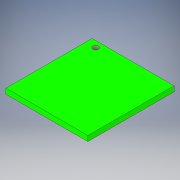
# Autodesk Inventor part: Vero_Board
Saved by Autodesk Inventor 2019.4 (Build 234330000, 330)
## iProperties
Created: 2021-06-29
Part Number: Vero_Board
Material: Generic
Document SubType Name: Modeling
Designer: keshav
Density: 1 g/cm^3
Appearance: Default
Author: keshav
Autodesk Inventor part; units mm, degrees
ref_plane "YZ Plane" through (0, 0, 0) normal (1, 0, 0) x (0, 1, 0)
ref_plane "XZ Plane" through (0, 0, 0) normal (0, 1, 0) x (-1, 0, 0)
ref_plane "XY Plane" through (0, 0, 0) normal (0, 0, 1) x (1, 0, 0)
sketch "Sketch1" plane through (0, 0, 0) normal (0, 1, 0) x (-1, 0, 0)
  line L0 (-12.5, 13.15) -> (12.5, 13.15)
  line L1 (12.5, 13.15) -> (12.5, -13.15)
  line L2 (12.5, -13.15) -> (-12.5, -13.15)
  line L3 (-12.5, -13.15) -> (-12.5, 13.15)
  line L4 (-12.5, 13.15) -> (12.5, -13.15) construction
  line L5 (12.5, 13.15) -> (-12.5, -13.15) construction
  circle A0 centre (9.475, -11.225) radius 0.85
  point P0 (0, 0)
  dimension "d0" = 25
  dimension "d1" = 26.3
  dimension "d2" = 1.7
  constraints: 12 end point, 2 midpoint, 2 parallel, 1 centre point, 1 horizontal, 1 perpendicular
  measures "d0" distance of L1.end L2.end
  measures "d1" distance of L0.end L1.end
  measures "d2" diameter of A0
extrude "Extrusion1" add sketch "Sketch1" along normal blind 1.6
body "Solid1"
